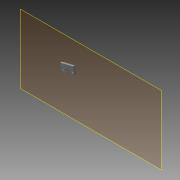
# Autodesk Inventor part: spacerBlock01
Saved by Autodesk Inventor 2013 (Build 170138000, 138)
## iProperties
Created: 2014-04-25
Part Number: spacerBlock01
Material: Generic
Document SubType Name: Modeling
Designer: Nano
Density: 1 g/cm^3
Author: Nano
Autodesk Inventor part; units mm, degrees
ref_plane "YZ Plane" through (0, 0, 0) normal (1, 0, 0) x (0, 1, 0)
ref_plane "XZ Plane" through (0, 0, 0) normal (0, 1, 0) x (-1, 0, 0)
ref_plane "XY Plane" through (0, 0, 0) normal (0, 0, 1) x (1, 0, 0)
ref_plane "Work Plane1" through (0, 0, 0) normal (0, 0, 1) x (1, 0, 0)
sketch "Sketch1" plane through (0, 0, 0) normal (0, 0, 1) x (1, 0, 0)
  circle A0 centre (-51.5287, 16.3728) radius 1.397 projected
  circle A1 centre (-33.9472, 20.9752) radius 1.397 projected
  line L0 (-56.5305, 24.9164) -> (-45.777, -18.2132) projected
  line L1 (-22.1173, -12.3142) -> (-32.8708, 30.8155) projected
  line L2 (-55.9143, 25.0701) -> (-33.4869, 30.6618)
  line L3 (-32.7171, 30.1993) -> (-29.7982, 18.4919)
  line L4 (-53.4579, 12.5929) -> (-56.3768, 24.3003)
  circle A2 centre (-42.2695, 18.1155) radius 1.5875 projected
  arc A3 (-37.6286, 19.1777) -> (-46.8891, 16.9637) centre (-42.2695, 18.1155) ccw
  line L5 (-42.2695, 18.1155) -> (-54.0994, 15.1659) construction
  line L6 (-46.8891, 16.9637) -> (-46.862, 16.8552)
  line L7 (-37.6509, 19.267) -> (-37.6238, 19.1585)
  line L8 (-30.2607, 17.7222) -> (-33.775, 16.8459)
  line L9 (-49.1746, 13.0064) -> (-52.6881, 12.1304)
  arc A4 (-49.1746, 13.0064) -> (-46.862, 16.8552) centre (-49.9427, 16.0871) ccw
  arc A5 (-37.6238, 19.1585) -> (-33.775, 16.8459) centre (-34.5431, 19.9266) ccw
  arc A6 (-55.9143, 25.0701) -> (-56.3768, 24.3003) centre (-55.7607, 24.4539) ccw
  arc A7 (-32.7171, 30.1993) -> (-33.4869, 30.6618) centre (-33.3333, 30.0457) ccw
  arc A8 (-53.4579, 12.5929) -> (-52.6881, 12.1304) centre (-52.8417, 12.7465) ccw
  arc A9 (-30.2607, 17.7222) -> (-29.7982, 18.4919) centre (-30.4143, 18.3383) ccw
  point P0 (0, 0)
  dimension "d0" = 3.175
  dimension "d1" = 0.635
  dimension "d2" = 0.635
  constraints: 16 end point, 14 point on circle, 12 tangent, 7 centre point, 5 parallel, 3 equal radius, 1 perpendicular, 1 point on line
  measures "d0" radius of A4
  measures "d1" radius of A6
  measures "d2" radius of A8
extrude "Extrusion1" add sketch "Sketch1" along normal blind 3.175 contours A6 L2 A7 L1 A9 L8 A5 L7 A3 L6 A4 L9 A8 L0
body "Solid1"
